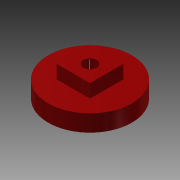
# Autodesk Inventor part: Tension Push washer backplate
Saved by Autodesk Inventor 2013 (Build 170138000, 138)
## iProperties
Created: 2012-11-15
Part Number: Tension Push washer backplate
Material: Generic
Document SubType Name: Modeling
Designer: Nico
Density: 1 g/cm^3
Author: Nico
Autodesk Inventor part; units mm, degrees
ref_plane "YZ Plane" through (0, 0, 0) normal (1, 0, 0) x (0, 1, 0)
ref_plane "XZ Plane" through (0, 0, 0) normal (0, 1, 0) x (-1, 0, 0)
ref_plane "XY Plane" through (0, 0, 0) normal (0, 0, 1) x (1, 0, 0)
sketch "Sketch1" plane through (0, 0, 0) normal (0, 0, 1) x (1, 0, 0)
  circle A0 centre (0, 0) radius 12.5
  dimension "d0" = 25
  constraints: 1 centre point, 1 coincident
  measures "d0" diameter of A0
extrude "Extrusion1" add sketch "Sketch1" along normal blind 5
sketch "Sketch2" plane through (0, 0, 5) normal (0, 0, 1) x (1, 0, 0)
  circle A0 centre (0, 0) radius 12.5 projected
  circle A1 centre (0, 0) radius 2
  dimension "d4" = 4
  constraints: 1 centre point, 1 coincident
  measures "d4" diameter of A1
extrude "Extrusion2" cut sketch "Sketch2" against normal blind 5 contours A1
sketch "Sketch3" plane through (0, 0, 5) normal (0, 0, 1) x (1, 0, 0)
  circle A0 centre (0, 0) radius 2 projected
  line L0 (-5, -5) -> (5, -5)
  line L1 (5, -5) -> (5, 5)
  line L2 (5, 5) -> (-5, 5)
  line L3 (-5, 5) -> (-5, -5)
  dimension "d8" = 10
  dimension "d10" = 10
  dimension "d11" = 5
  dimension "d12" = 5
  constraints: 8 end point, 2 parallel, 1 horizontal, 1 perpendicular
  measures "d8" distance of L1.end L2.end
  measures "d10" distance between parallel lines of L0 L2
  measures "d11" distance from line of A0.centre L2
  measures "d12" distance from line of A0.centre L1
extrude "Extrusion3" add sketch "Sketch3" along normal blind 4
sketch "Sketch4" plane through (0, 0, 0) normal (0, 0, -1) x (-1, 0, 0)
  circle A0 centre (0, 0) radius 2 projected
  circle A1 centre (0, 0) radius 12.5 projected
  line L0 (-2.023, 3.4987) -> (2.0185, 3.5013)
  line L1 (2.0185, 3.5013) -> (4.0415, 0.0026)
  line L2 (4.0415, 0.0026) -> (2.023, -3.4987)
  line L3 (2.023, -3.4987) -> (-2.0185, -3.5013)
  line L4 (-2.0185, -3.5013) -> (-4.0415, -0.0026)
  line L5 (-4.0415, -0.0026) -> (-2.023, 3.4987)
  dimension "d15" = 7
  constraints: 12 end point, 1 coincident, 13 other
  measures "d15" distance between parallel lines of L3 L0
extrude "Extrusion4" cut sketch "Sketch4" against normal blind 4 contours L0 L1 L2 L3 L4 L5
body "Solid1"
